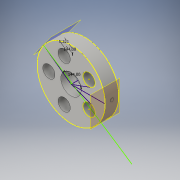
# Autodesk Inventor part: Flansch
Saved by Autodesk Inventor 2016 (Build 200138000, 138)
## iProperties
Created: 2017-12-01
Part Number: Flansch
Material: Generisch
Document SubType Name: Modeling
Designer: Dominik
Density: 1 g/cm^3
Appearance: Vorgabe
Author: Dominik
Autodesk Inventor part; units mm, degrees
ref_plane "YZ Plane" through (0, 0, 0) normal (1, 0, 0) x (0, 1, 0)
ref_plane "XZ Plane" through (0, 0, 0) normal (0, 1, 0) x (-1, 0, 0)
ref_plane "XY Plane" through (0, 0, 0) normal (0, 0, 1) x (1, 0, 0)
sketch "Skizze1" plane through (0, 0, 0) normal (0, 1, 0) x (-1, 0, 0)
  circle A0 centre (0, 0) radius 7.5
  circle A1 centre (0, 0) radius 25
  dimension "d0" = 15
  dimension "d1" = 50
  constraints: 2 centre point, 2 coincident
  measures "d0" diameter of A0
  measures "d1" diameter of A1
extrude "Extrusion1" add sketch "Skizze1" along normal blind 10
sketch "Skizze2" plane through (0, 10, 0) normal (0, 1, 0) x (1, 0, 0)
  circle A0 centre (0, 0) radius 25 projected
  line L0 (-25, 0) -> (-16.25, 0)
  line L1 (0, 0) -> (8.75, 0) construction
  line L2 (0, 0) -> (-5.0215, 15.4547)
  line L3 (0, 0) -> (16.25, 0) construction
  line L4 (0, 0) -> (13.1465, 9.5515)
  line L5 (0, 0) -> (16.25, 0) construction
  line L6 (0, 0) -> (16.25, 0) construction
  line L7 (0, 0) -> (13.1465, -9.5515)
  line L8 (0, 0) -> (16.25, 0) construction
  line L9 (0, 0) -> (-5.0215, -15.4547)
  line L10 (0, 0) -> (16.25, 0) construction
  circle A1 centre (-16.25, 0) radius 4.3
  circle A2 centre (-5.0215, 15.4547) radius 4.3
  circle A3 centre (13.1465, 9.5515) radius 4.3
  circle A4 centre (13.1465, -9.5515) radius 4.3
  circle A5 centre (-5.0215, -15.4547) radius 4.3
  dimension "d4" = 8.75
  dimension "d9" = 16.25
  dimension "d10" = 108
  dimension "d11" = 16.25
  dimension "d12" = 36
  dimension "d15" = 16.25
  dimension "d16" = 36
  dimension "d17" = 16.25
  dimension "d18" = 108
  dimension "d19" = 8.6
  dimension "d20" = 8.6
  dimension "d21" = 8.6
  dimension "d22" = 8.6
  dimension "d23" = 8.6
  constraints: 22 end point, 7 horizontal, 5 centre point, 5 coincident, 4 equal length, 1 horizontal alignment, 1 other
  measures "d4" distance of L0.start L0.end
  measures "d9" distance of L1.start L2.end
  measures "d10" angle of L3 L2
  measures "d11" distance of L1.start L4.end
  measures "d12" angle of L5 L4
  measures "d15" distance of L1.start L7.end
  measures "d16" angle of L7 L8
  measures "d17" distance of L1.start L9.end
  measures "d18" angle of L9 L10
  measures "d19" diameter of A1
  measures "d20" diameter of A2
  measures "d21" diameter of A3
  measures "d22" diameter of A4
  measures "d23" diameter of A5
hole "Bohrung1" at (-16.25, 10, 0) at (-5.0215, 10, -15.4547) at (13.1465, 10, -9.5515) at (13.1465, 10, 9.5515) at (-5.0215, 10, 15.4547) direction (0, -1, 0) diameter 9 end through all
sketch "Skizze3" plane through (0, 0, 0) normal (1, 0, 0) x (0, 1, 0)
  point P0 (0, 0)
sketch "Skizze4" plane through (0, 0, 0) normal (1, 0, 0) x (0, 1, 0)
  line L0 (0, 0) -> (5, 0)
  constraints: 2 end point, 1 horizontal
sketch "Skizze6" plane through (0, 10, 0) normal (0, 1, 0) x (1, 0, 0)
  circle A0 centre (-5.0215, -15.4547) radius 4.5 projected
  circle A1 centre (-16.25, 0) radius 4.5 projected
  circle A2 centre (0, 0) radius 25 projected
  line L0 (0, 0) -> (-8.7488, -12.9333)
  line L1 (0, 0) -> (-15.0038, -4.324)
  line L2 (-11.8428, -8.6043) -> (-20.2254, -14.6946)
  line L3 (-11.8428, -8.6043) -> (-1.4813, -8.6043) construction
  line L4 (0, 0) -> (-11.8428, -8.6043)
  dimension "d36" = 5.321
  dimension "d37" = 144
  constraints: 10 end point, 1 collinear, 1 equal length, 1 horizontal, 8 other
  measures "d36" distance of L0.end L2.start
  measures "d37" angle of L2 L3
sketch "Skizze7" plane through (0, 0, 0) normal (0, -1, 0) x (1, 0, 0)
  line L0 (0, 0) -> (-20.2254, 14.6946)
  circle A0 centre (0, 0) radius 25 projected
  line L1 (0, 0) -> (25, 0) construction
  line L2 (-20.2254, 14.6946) -> (44.6167, -28.5072)
  dimension "d38" = 144
  constraints: 6 end point, 1 equal length, 1 horizontal, 2 other
  measures "d38" angle of L1 L0
ref_plane "Arbeitsebene1" through (-20.2254, 10, 14.6946) normal (-0.809017, 0, 0.5877853) x (0, -1, 0)
sketch "Skizze8" plane through (-20.2254, 10, 14.6946) normal (-0.809017, 0, 0.5877853) x (0, -1, 0)
  line L0 (10, 0) -> (5, 0)
  dimension "d39" = 5
  constraints: 2 end point, 1 horizontal
  measures "d39" distance of L0.start L0.end
hole "Bohrung2" at (-20.2254, 5, 14.6946) direction (0.809017, 0, -0.5877853) diameter 2.459 depth 27.8 tip angle 118 thread size "M3x0.5" class "6H" standard "ISO Metric profile"
sketch "Skizze9" plane through (0, 0, 0) normal (0, -1, 0) x (1, 0, 0)
  line L0 (0, 0) -> (25, 0)
  circle A0 centre (0, 0) radius 25 projected
  line L1 (0, 0) -> (14.68, 5.3208)
  circle A1 centre (13.1465, 9.5515) radius 4.5 projected
  line L2 (0, 0) -> (14.68, -5.3208)
  circle A2 centre (13.1465, -9.5515) radius 4.5 projected
  line L3 (0, 0) -> (25, 0)
  constraints: 8 end point, 1 collinear, 1 horizontal, 1 horizontal alignment, 7 other
sketch "Skizze10" plane through (0, 10, 0) normal (0, 1, 0) x (1, 0, 0)
  line L0 (0, 0) -> (25, 0)
  circle A0 centre (0, 0) radius 25 projected
  constraints: 2 end point, 1 horizontal, 1 horizontal alignment, 1 other
ref_plane "Arbeitsebene2" through (25, 0, 0) normal (1, 0, 0) x (0, 1, 0)
sketch "Skizze11" plane through (25, 0, 0) normal (1, 0, 0) x (0, 1, 0)
  line L0 (0, 0) -> (5, 0)
  dimension "d47" = 5
  constraints: 2 end point, 1 horizontal
  measures "d47" distance of L0.start L0.end
hole "Bohrung3" at (25, 5, 0) direction (-1, 0, 0) diameter 2.459 depth 27.8 tip angle 118 thread size "M3x0.5" class "6H" standard "ISO Metric profile"
